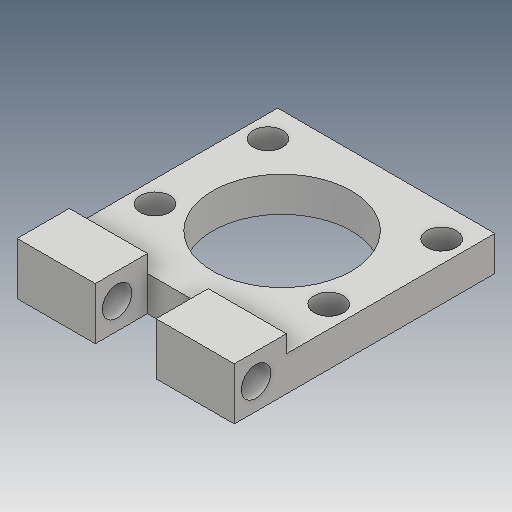
# Autodesk Inventor part: kamera ot
Saved by Autodesk Inventor 2018 (Build 220112000, 112)
## iProperties
Created: 2018-01-30
Part Number: kamera ot
Material: Generisch
Document SubType Name: Modeling
Designer: Andreas
Density: 1 g/cm^3
Appearance: Vorgabe
Mass: 1.93506 g
Surface Area: 20.7716 cm^2
Volume: 1.93506 cm^3
Author: Andreas
Autodesk Inventor part; units mm, degrees
ref_plane "YZ Plane" through (0, 0, 0) normal (1, 0, 0) x (0, 1, 0)
ref_plane "XZ Plane" through (0, 0, 0) normal (0, 1, 0) x (-1, 0, 0)
ref_plane "XY Plane" through (0, 0, 0) normal (0, 0, 1) x (1, 0, 0)
sketch "Skizze1" plane through (0, 0, 0) normal (0, 0, 1) x (1, 0, 0)
  line L0 (0, 0) -> (25, 0)
  line L1 (25, 0) -> (25, 30)
  line L2 (25, 30) -> (0, 30)
  line L3 (0, 30) -> (0, 0)
  dimension "d0" = 30
  dimension "d1" = 25
  constraints: 8 end point, 2 parallel, 1 horizontal, 1 perpendicular
  measures "d0" distance of L0.end L1.end
  measures "d1" distance of L1.end L2.end
extrude "Extrusion1" add sketch "Skizze1" against normal blind 6
sketch "Skizze2" plane through (0, 0, 0) normal (0, 0, 1) x (1, 0, 0)
  circle A0 centre (12.5, 18) radius 8
  line L0 (25, 0) -> (25, 30) projected
  line L1 (0, 0) -> (25, 0) projected
  dimension "d4" = 16
  dimension "d5" = 12.5
  dimension "d6" = 18
  constraints: 1 centre point
  measures "d4" diameter of A0
  measures "d5" distance from line of L0 A0.centre
  measures "d6" distance from line of L1 A0.centre
extrude "Extrusion2" cut sketch "Skizze2" against normal blind 10
sketch "Skizze4" plane through (0, 0, 0) normal (0, 0, 1) x (1, 0, 0)
  line L0 (2.5, 13.3758) -> (22.5, 13.3758) construction
  line L1 (22.5, 13.3758) -> (22.5, 26.3758) construction
  line L2 (22.5, 26.3758) -> (2.5, 26.3758) construction
  line L3 (2.5, 26.3758) -> (2.5, 13.3758) construction
  line L4 (25, 0) -> (25, 30) construction
  circle A0 centre (2.5, 26.3758) radius 1.7
  circle A1 centre (22.5, 26.3758) radius 1.7
  circle A2 centre (22.5, 13.3758) radius 1.7
  circle A3 centre (2.5, 13.3758) radius 1.7
  point P0 (0, 0)
  point P1 (25, 3.0001)
  dimension "d12" = 20
  dimension "d13" = 13
  dimension "d14" = 2.5
  dimension "d15" = 3.4
  dimension "d16" = 3.4
  dimension "d17" = 3.4
  dimension "d18" = 3.4
  constraints: 8 end point, 4 centre point, 4 coincident, 2 parallel, 1 horizontal, 1 perpendicular
  measures "d12" distance of L1.end L2.end
  measures "d13" distance of L2.end L0.start
  measures "d14" distance between parallel lines of L4 L1
  measures "d15" diameter of A0
  measures "d16" diameter of A1
  measures "d17" diameter of A2
  measures "d18" diameter of A3
extrude "Extrusion4" cut sketch "Skizze4" against normal blind 10
sketch "Skizze6" plane through (0, 0, 0) normal (0, 0, 1) x (1, 0, 0)
  line L0 (25, 0) -> (0, 0) projected
  line L1 (25, 0) -> (16, 0)
  line L2 (16, 0) -> (16, 6)
  line L3 (16, 6) -> (25, 6)
  line L4 (25, 6) -> (25, 0)
  line L5 (0, 0) -> (9, 0)
  line L6 (9, 0) -> (9, 6)
  line L7 (9, 6) -> (0, 6)
  line L8 (0, 6) -> (0, 0)
  line L9 (9, 6) -> (16, 6)
  line L10 (16, 6) -> (16, 0)
  line L11 (16, 0) -> (9, 0)
  line L12 (9, 0) -> (9, 6)
  dimension "d21" = 9
  dimension "d22" = 9
  dimension "d23" = 6
  constraints: 24 end point, 6 parallel, 3 horizontal, 3 perpendicular, 1 point on line
  measures "d21" distance of L6.end L7.end
  measures "d22" distance of L2.end L3.end
  measures "d23" distance of L5.end L6.end
extrude "Extrusion5" cut sketch "Skizze6" against normal blind 10 contours L0 L6 L9 L2
sketch "Skizze7" plane through (0, 0, 0) normal (-1, 0, 0) x (0, 0, 1)
  circle A0 centre (-3, 2.5) radius 1.7
  line L0 (0, 30) -> (0, 0) projected
  line L1 (0, 0) -> (-6, 0) projected
  dimension "d26" = 3.4
  dimension "d27" = 3
  dimension "d28" = 2.5
  constraints: 1 centre point
  measures "d26" diameter of A0
  measures "d27" distance from line of L0 A0.centre
  measures "d28" distance from line of L1 A0.centre
extrude "Extrusion6" cut sketch "Skizze7" against normal blind 40
sketch "Skizze8" plane through (0, 0, 0) normal (0, 0, 1) x (1, 0, 0)
  line L0 (16, 6) -> (16, 0) projected
  line L1 (16, 0) -> (25, 0) projected
  line L2 (25, 0) -> (25, 30) projected
  line L3 (25, 30) -> (0, 30) projected
  line L4 (0, 30) -> (0, 0) projected
  line L5 (0, 0) -> (9, 0) projected
  line L6 (9, 0) -> (9, 6) projected
  line L7 (9, 6) -> (16, 6) projected
  circle A0 centre (22.5, 13.3758) radius 1.7 projected
  circle A1 centre (2.5, 26.3758) radius 1.7 projected
  circle A2 centre (22.5, 26.3758) radius 1.7 projected
  circle A3 centre (2.5, 13.3758) radius 1.7 projected
  circle A4 centre (12.5, 18) radius 8 projected
  line L8 (0, 30) -> (0, 0) projected
  line L9 (0, 6) -> (25, 6)
  line L10 (25, 0) -> (25, 30) projected
  line L11 (25, 6) -> (25, 30)
  line L12 (25, 30) -> (0, 30) projected
  line L13 (25, 30) -> (0, 30)
  line L14 (0, 30) -> (0, 6)
  constraints: 8 end point, 3 collinear, 3 point on line
extrude "Extrusion7" cut sketch "Skizze8" against normal blind 2 contours L7 L9 L4 L3 L2
